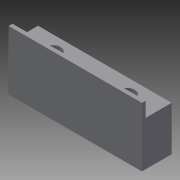
# Autodesk Inventor part: Slider
Saved by Autodesk Inventor 2015 (Build 190159000, 159)
## iProperties
Created: 2016-05-27
Part Number: Slider
Material: Generic
Document SubType Name: Modeling
Designer: Toby
Density: 1 g/cm^3
Appearance: Default
Author: Toby
Autodesk Inventor part; units mm, degrees
ref_plane "YZ Plane" through (0, 0, 0) normal (1, 0, 0) x (0, 1, 0)
ref_plane "XZ Plane" through (0, 0, 0) normal (0, 1, 0) x (-1, 0, 0)
ref_plane "XY Plane" through (0, 0, 0) normal (0, 0, 1) x (1, 0, 0)
sketch "Sketch1" plane through (0, 0, 0) normal (0, 0, 1) x (1, 0, 0)
  line L0 (-18.0312, 10.7455) -> (26.9688, 10.7455)
  line L1 (26.9688, 10.7455) -> (26.9688, 0.7455)
  line L2 (26.9688, 0.7455) -> (-18.0312, 0.7455)
  line L3 (-18.0312, 0.7455) -> (-18.0312, 10.7455)
  circle A0 centre (-8.0312, 5.7455) radius 2.6
  circle A1 centre (16.9688, 5.7455) radius 2.6
  point P0 (0, 0)
  dimension "d0" = 5.2
  dimension "d1" = 5.2
  dimension "d2" = 10
  dimension "d3" = 5
  dimension "d4" = 5
  dimension "d5" = 10
  dimension "d6" = 45
  dimension "d7" = 10
  dimension "d8" = 25
  constraints: 8 end point, 2 centre point, 2 parallel, 1 horizontal, 1 perpendicular
  measures "d0" diameter of A0
  measures "d1" diameter of A1
  measures "d2" distance of L2.end L0.start
  measures "d3" distance from line of L0 A0.centre
  measures "d4" distance from line of A1.centre L0
  measures "d5" distance from line of L3 A0.centre
  measures "d6" distance of L0.start L0.end
  measures "d7" distance from line of L1 A1.centre
  measures "d8" distance of A1.centre A0.centre
extrude "Extrusion1" add sketch "Sketch1" along normal blind 15
sketch "Sketch2" plane through (0, 0, 15) normal (0, 0, 1) x (1, 0, 0)
  line L0 (-17.927, 2.0194) -> (26.9688, 2.0194)
  line L1 (26.9688, 2.0194) -> (26.9688, 0.7455)
  line L2 (26.9688, 0.7455) -> (-17.927, 0.7455)
  line L3 (-17.927, 0.7455) -> (-17.927, 2.0194)
  point P0 (0, 0)
  constraints: 8 end point, 2 parallel, 1 horizontal, 1 perpendicular
extrude "Extrusion2" add sketch "Sketch2" along normal blind 5
body "Solid1"
